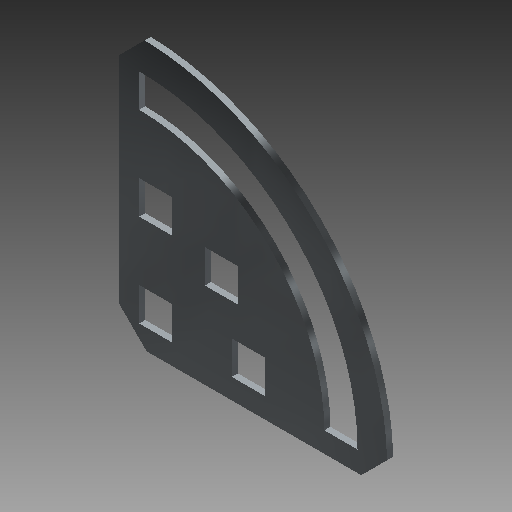
# Autodesk Inventor part: 275-1062
Saved by Autodesk Inventor 2018 (Build 220112000, 112)
## iProperties
Company: Autodesk Inc.
Category: Structure
Created: 2012-04-11
Part Number: 275-1062
Document SubType Name: Modeling
Designer: Autodesk Inc.
Density: 7.85 g/cm^3
Catalog Web Link: http://www.vexrobotics.com/products/accessories/structure/275-1062.html
Vendor: VEX
Material: Steel
Mass: 5.30008 g
Surface Area: 18.5876 cm^2
Volume: 0.67517 cm^3
Appearance: Zinc
Author: Autodesk Inc.
Autodesk Inventor part; units mm, degrees
ref_plane "YZ Plane" through (0, 0, 0) normal (1, 0, 0) x (0, 1, 0)
ref_plane "XZ Plane" through (0, 0, 0) normal (0, 1, 0) x (-1, 0, 0)
ref_plane "XY Plane" through (0, 0, 0) normal (0, 0, 1) x (1, 0, 0)
sketch "Sketch1" plane through (0, 0, 0) normal (0, 0, 1) x (1, 0, 0)
  line L0 (-25.4584, -1.6339) -> (-20.8864, -1.6339)
  line L1 (-20.8864, -1.6339) -> (-20.8864, -6.2059)
  line L2 (-20.8864, -6.2059) -> (-25.4584, -6.2059)
  line L3 (-25.4584, -6.2059) -> (-25.4584, -1.6339)
  line L4 (-12.7584, -6.2059) -> (-8.1864, -6.2059)
  line L5 (-8.1864, -6.2059) -> (-8.1864, -1.6339)
  line L6 (-8.1864, -1.6339) -> (-12.7584, -1.6339)
  line L7 (-12.7584, -1.6339) -> (-12.7584, -6.2059)
  line L8 (-0.0584, -6.2059) -> (4.5136, -6.2059)
  line L9 (-25.4584, 6.4941) -> (-20.8864, 6.4941)
  line L10 (-20.8864, 6.4941) -> (-20.8864, 11.0661)
  line L11 (-20.8864, 11.0661) -> (-25.4584, 11.0661)
  line L12 (-25.4584, 11.0661) -> (-25.4584, 6.4941)
  line L13 (-25.4584, 23.7661) -> (-25.4584, 19.1941)
  line L14 (-24.4424, -8.9999) -> (5.0216, -8.9999)
  line L15 (-28.2524, -5.1899) -> (-28.2524, 24.2741)
  arc A0 (-0.0584, -6.2059) -> (-25.4584, 19.1941) centre (-25.4584, -6.2059) ccw
  arc A1 (4.5136, -6.2059) -> (-25.4584, 23.7661) centre (-25.4584, -6.2059) ccw
  arc A2 (8.5693, -5.4523) -> (-24.7047, 27.8217) centre (-25.4584, -6.2059) ccw
  line L16 (-28.2524, -5.1899) -> (-24.4424, -8.9999)
  line L17 (-24.4424, -8.9999) -> (-28.2524, -5.1899)
  line L18 (-28.2524, 24.2741) -> (-24.7047, 27.8217)
  line L19 (8.5693, -5.4523) -> (5.0216, -8.9999)
  line L20 (-16.4414, 2.8111) -> (-11.8694, 2.8111)
  line L21 (-11.8694, 2.8111) -> (-11.8694, 7.3831)
  line L22 (-11.8694, 7.3831) -> (-16.4414, 7.3831)
  line L23 (-16.4414, 7.3831) -> (-16.4414, 2.8111)
  point P0 (-28.2524, -8.9999)
  point P1 (-28.2524, -8.9999)
  dimension "d0" = 4.572
  dimension "d1" = 4.572
  dimension "d2" = 4.572
  dimension "d3" = 4.572
  dimension "d4" = 4.572
  dimension "d5" = 4.572
  dimension "d6" = 8.128
  dimension "d8" = 8.128
  dimension "d10" = 4.064
  dimension "d11" = 2.794
  dimension "d12" = 2.794
  dimension "d13" = 3.81
  dimension "d14" = 3.81
  dimension "d15" = 3.81
  dimension "d16" = 3.81
  dimension "d18" = 45
  dimension "d22" = 4.572
  dimension "d23" = 4.445
  dimension "d24" = 4.445
  dimension "d25" = 4.572
  constraints: 48 end point, 8 parallel, 6 perpendicular, 6 point on circle, 6 point on line, 5 collinear, 5 horizontal, 3 centre point, 3 coincident
  measures "d0" distance of L1.end L2.end
  measures "d1" distance of L0.end L1.end
  measures "d2" distance of L4.start L4.end
  measures "d3" distance of L8.start L8.end
  measures "d4" distance of L11.end L9.start
  measures "d5" distance of L13.start L13.end
  measures "d6" distance between parallel lines of L9 L0
  measures "d8" distance between parallel lines of L7 L1
  measures "d10" radial gap between concentric circles of A2 A1
  measures "d11" distance between parallel lines of L14 L2
  measures "d12" distance between parallel lines of L15 L3
  measures "d13" distance of L16.start point (-28.252, -9)
  measures "d14" distance of L16.end point (-28.252, -9)
  measures "d15" distance of L14.start point (-28.252, -9)
  measures "d16" distance of L15.start point (-28.252, -9)
  measures "d18" angle of L15 L18
  measures "d22" distance of L20.start L20.end
  measures "d23" distance between parallel lines of L6 L20
  measures "d24" distance between parallel lines of L23 L10
  measures "d25" distance between parallel lines of L22 L20
extrude "Extrusion1" add sketch "Sketch1" along normal blind 0.8382
sketch "Sketch2" plane through (0, 0, 0.8382) normal (0, 0, 1) x (1, 0, 0)
  line L0 (-20.8864, -1.6339) -> (-20.8864, -6.2059) projected
  line L1 (-20.8864, -6.2059) -> (-25.4584, -6.2059) projected
  line L2 (-25.4584, -6.2059) -> (-25.4584, -1.6339) projected
  line L3 (-25.4584, -1.6339) -> (-20.8864, -1.6339) projected
  circle A0 centre (-23.1724, -3.9199) radius 2.286
  point P0 (0, 0)
  constraints: 4 tangent, 1 centre point
surface extrude "ExtrusionSrf1" sketch "Sketch2" against normal up to surface (0.8382 mm away) shown no curves A0
pattern_linear "Rectangular Pattern1" count 2 spacing 12.7 along (1, 0, 0) of "ExtrusionSrf1"
pattern_linear "Rectangular Pattern2" count 2 spacing 12.7 along (0, 1, 0) of "ExtrusionSrf1"
sketch "Sketch3" plane through (0, 0, 0.8382) normal (0, 0, 1) x (1, 0, 0)
  line L0 (-16.4414, 2.8111) -> (-16.4414, 7.3831) projected
  line L1 (-16.4414, 7.3831) -> (-11.8694, 7.3831) projected
  line L2 (-11.8694, 7.3831) -> (-11.8694, 2.8111) projected
  line L3 (-11.8694, 2.8111) -> (-16.4414, 2.8111) projected
  circle A0 centre (-14.1554, 5.0971) radius 2.286
  point P0 (0, 0)
  constraints: 4 tangent, 1 centre point
surface extrude "ExtrusionSrf4" sketch "Sketch3" against normal up to surface (0.8382 mm away) shown no curves A0
sketch "Sketch4" plane through (0, 0, 0.8382) normal (0, 0, 1) x (1, 0, 0)
  arc A0 (-0.0584, -6.2059) -> (-25.4584, 19.1941) centre (-25.4584, -6.2059) ccw projected
  line L0 (-25.4584, 19.1941) -> (-25.4584, 23.7661) projected
  arc A1 (4.5136, -6.2059) -> (-25.4584, 23.7661) centre (-25.4584, -6.2059) ccw projected
  circle A2 centre (-23.1724, 21.3855) radius 2.286
  point P0 (0, 0)
  constraints: 3 tangent, 1 centre point
surface extrude "ExtrusionSrf5" sketch "Sketch4" against normal up to surface (0.8382 mm away) shown no curves A2
sketch "Sketch5" plane through (0, 0, 0.8382) normal (0, 0, 1) x (1, 0, 0)
  arc A0 (-0.0584, -6.2059) -> (-25.4584, 19.1941) centre (-25.4584, -6.2059) ccw projected
  arc A1 (4.5136, -6.2059) -> (-25.4584, 23.7661) centre (-25.4584, -6.2059) ccw projected
  line L0 (4.5136, -6.2059) -> (-0.0584, -6.2059) projected
  circle A2 centre (2.1331, -3.9199) radius 2.286
  point P0 (0, 0)
  constraints: 3 tangent, 1 centre point
surface extrude "ExtrusionSrf6" sketch "Sketch5" against normal up to surface (0.8382 mm away) shown no curves A2
equation "\"d14\" = d13"
equation "\"d15\" = d13"
equation "\"d16\" = d15"
body "Solid1"
body "Srf1"
body "Srf2"
body "Srf3"
body "Srf4"
body "Srf5"
body "Srf6"
